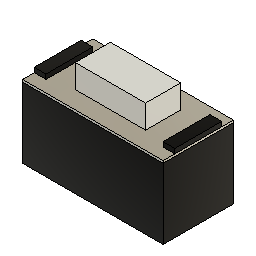
3dmodel_20240416 (Autodesk Fusion 360 archive; units mm, degrees)
design "SW_タクト"
Autodesk Fusion 360 part; units mm, degrees
sketch "スケッチ1" plane through (0, 0, 0) normal (0, 0, 1) x (1, 0, 0)
  line L0 (3, 1.5) -> (-3, 1.5)
  line L1 (-3, 1.5) -> (-3, -1.5)
  line L2 (-3, -1.5) -> (3, -1.5)
  line L3 (3, -1.5) -> (3, 1.5)
  line L4 (3, 1.5) -> (-3, -1.5) construction
  line L5 (-3, 1.5) -> (3, -1.5) construction
  dimension "d1" = 6
  dimension "d2" = 3
  constraint horizontal L0
  constraint perpendicular L0 L1
  constraint parallel L0 L2
  constraint parallel L1 L3
  constraint coincident L4 origin
  constraint coincident L5 origin
  measures "d1" distance of L1.end L2.end
  measures "d2" distance of L0.end L1.end
extrude "押し出し1" add sketch "スケッチ1" along normal blind 3 makes body 1
sketch "スケッチ2" plane through (0, 0, 3) normal (0, 0, 1) x (-1, 0, 0)
  line L0 (-3, 1.5) -> (-3, -1.5)
  line L1 (-3, -1.5) -> (3, -1.5)
  line L2 (3, -1.5) -> (3, 1.5)
  line L3 (3, 1.5) -> (-3, 1.5)
extrude "押し出し2" add sketch "スケッチ2" along normal blind 0.1 separate body makes body 2
sketch "スケッチ3" plane through (0, 0, 3.1) normal (0, 0, 1) x (-1, 0, 0)
  line L0 (3, 1.5) -> (-3, 1.5)
  line L1 (-3, 1.5) -> (-3, -1.5)
  line L2 (-3, -1.5) -> (3, -1.5)
  line L3 (3, -1.5) -> (3, 1.5)
  line L4 (-1.5, 0.75) -> (1.5, 0.75)
  line L5 (1.5, 0.75) -> (1.5, -0.75)
  line L6 (1.5, -0.75) -> (-1.5, -0.75)
  line L7 (-1.5, -0.75) -> (-1.5, 0.75)
  line L8 (-1.5, 0.75) -> (1.5, -0.75) construction
  line L9 (1.5, 0.75) -> (-1.5, -0.75) construction
  line L10 (3, 0) -> (3, -1)
  line L11 (3, -1) -> (2.5, -1)
  line L12 (2.5, -1) -> (2.5, 1)
  line L13 (2.5, 1) -> (3, 1)
  line L14 (3, 0) -> (3, 1)
  line L15 (-3, 0) -> (-3, 1)
  line L16 (-3, 0) -> (-3, -1)
  line L17 (-3, -1) -> (-2.5, -1)
  line L18 (-2.5, 1) -> (-3, 1)
  line L19 (-2.5, -1) -> (-2.5, 1)
  dimension "d7" = 3
  dimension "d8" = 1.5
  dimension "d11" = 1
  dimension "d12" = 0.5
  dimension "d13" = 2
  constraint horizontal L4
  constraint perpendicular L4 L5
  constraint parallel L4 L6
  constraint parallel L5 L7
  constraint coincident L8 origin
  constraint coincident L9 origin
  constraint midpoint L3 L10.start
  constraint parallel L3 L10
  constraint perpendicular L10 L11
  constraint perpendicular L11 L12
  constraint perpendicular L12 L13
  constraint perpendicular L13 L14
  measures "d7" distance of L5.end L6.end
  measures "d8" distance of L4.end L5.end
  measures "d11" distance of L10.start L10.end
  measures "d12" distance of L10.end L11.end
  measures "d13" distance of L11.end L12.end
extrude "押し出し3" add sketch "スケッチ3" along normal blind 1 separate body contours L4 L5 L6 L7 makes body 3
extrude "押し出し4" add sketch "スケッチ3" along normal blind 0.2 separate body contours L3 L10 L11 L12 L13 L14 | L1 L15 L16 L17 L18 L19 makes body 4 at (-2.6667, -0.3333, 3.1) makes body 5 at (2.8333, -0.3333, 3.1)

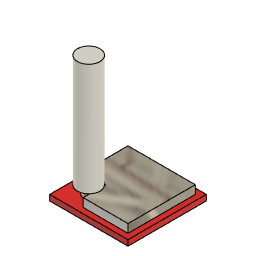
design "TWE-Lite-RED"
Autodesk Fusion 360 part; units mm, degrees
sketch "スケッチ1" plane through (0, 0, 0) normal (0, 0, 1) x (1, 0, 0)
  line L0 (6.985, -6.985) -> (-6.985, -6.985)
  line L1 (-6.985, -6.985) -> (-6.985, 6.985)
  line L2 (-6.985, 6.985) -> (6.985, 6.985)
  line L3 (6.985, 6.985) -> (6.985, -6.985)
  line L4 (6.985, -6.985) -> (-6.985, 6.985) construction
  line L5 (-6.985, -6.985) -> (6.985, 6.985) construction
  dimension "d1" = 13.97
  dimension "d2" = 13.97
  constraint horizontal L0
  constraint perpendicular L0 L1
  constraint parallel L0 L2
  constraint parallel L1 L3
  constraint coincident L4 origin
  constraint coincident L5 origin
  measures "d1" distance of L1.end L2.end
  measures "d2" distance of L0.end L1.end
extrude "押し出し1" add sketch "スケッチ1" along normal blind 1 makes body 1
sketch "スケッチ2" plane through (0, 0, 1) normal (0, 0, 1) x (-1, 0, 0)
  line L0 (-6.985, -6.985) -> (6.985, -6.985)
  line L1 (6.985, -6.985) -> (6.985, 6.985)
  line L2 (6.985, 6.985) -> (-6.985, 6.985)
  line L3 (-6.985, 6.985) -> (-6.985, -6.985)
  line L4 (6, 6) -> (-6, 6)
  line L5 (-6, 6) -> (-6, -6)
  line L6 (-6, -6) -> (6, -6)
  line L7 (6, -6) -> (6, 6)
  line L8 (6, 6) -> (2, 6)
  line L9 (2, 6) -> (2, 2)
  line L10 (2, 2) -> (6, 2)
  line L11 (6, 2) -> (6, 6)
  circle A0 centre (3.5, 3.5) radius 1
  circle A1 centre (3.5, 3.5) radius 0.9
  dimension "d5" = 12
  dimension "d6" = 12
  dimension "d7" = 4
  dimension "d8" = 4
  dimension "d13" = 2
  dimension "d14" = -0.1
  constraint horizontal L4
  constraint perpendicular L4 L5
  constraint parallel L4 L6
  constraint parallel L5 L7
  constraint horizontal L8
  constraint vertical L9
  constraint horizontal L10
  constraint vertical L11
  measures "d5" distance of L5.end L6.end
  measures "d6" distance of L4.end L5.end
  measures "d7" distance of L4.start L8.end
  measures "d8" distance of L4.start L10.end
  measures "d13" diameter of A0
extrude "押し出し2" add sketch "スケッチ2" along normal blind 1.5 separate body contours L4 L5 L6 L7 L9 L10 makes body 2
extrude "押し出し3" add sketch "スケッチ2" along normal blind 1.5 separate body contours A0 makes body 3
sketch "スケッチ3" plane through (0, 0, 2.5) normal (0, 0, 1) x (-1, 0, 0)
  circle A0 centre (3.5, 3.5) radius 0.9
  circle A1 centre (3.5, 3.5) radius 1
  circle A2 centre (3.5, 3.5) radius 2
  dimension "d17" = 4
  constraint concentric A0 A2
  measures "d17" diameter of A2
extrude "押し出し4" add sketch "スケッチ3" along normal blind 20 separate body contours A0 | A1 | A2 makes body 4
